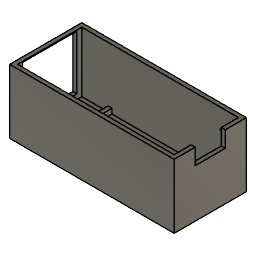
lensdisplayModule (Autodesk Fusion 360 design; units mm, degrees)
part number: 2026-07-30-17-18-59-911
part number: 2026-07-30-18-52-39-919
Autodesk Fusion 360 part; units mm, degrees
sketch "Sketch1" plane through (0, 0, 0) normal (0, 1, 0) x (1, 0, 0) in component "Display_Lens"
sketch "Sketch2" plane through (0, 0, 0) normal (0, 0, 1) x (1, 0, 0) in component "Display_Lens"
  line L0 (0, 0) -> (82, 0)
  line L1 (82, 0) -> (82, 36)
  line L2 (82, 36) -> (0, 36)
  line L3 (0, 36) -> (0, 0)
  dimension "d1" = 82
  dimension "d2" = 36
  constraint horizontal L0
  constraint vertical L1
  constraint horizontal L2
  constraint vertical L3
  constraint coincident L0.start L3.end
  measures "d1" distance of L0.start L0.end
  measures "d2" distance of L0.start L2.end
extrude "ExtrudedCentralBase" add sketch "Sketch2" along normal blind 34 in component "Display_Lens"
shell "Removed2mmTop" thickness 2 removed faces 1 at (27.3333, 24, 34) in component "Display_Lens"
sketch "CreatedLensViewWindow" plane through (2, 0, 0) normal (1, 0, 0) x (0, 1, 0) in component "Display_Lens"
  line L0 (2, 2) -> (34, 2)
  line L1 (34, 2) -> (34, 34)
  line L2 (34, 34) -> (2, 34)
  line L3 (2, 34) -> (2, 2)
  line L4 (4.5, 31.5) -> (31.5, 31.5)
  line L5 (31.5, 31.5) -> (31.5, 4.5)
  line L6 (31.5, 4.5) -> (4.5, 4.5)
  line L7 (4.5, 4.5) -> (4.5, 31.5)
  line L8 (4.5, 31.5) -> (31.5, 4.5) construction
  line L9 (31.5, 31.5) -> (4.5, 4.5) construction
  point P0 (18, 18)
  dimension "d8" = 27
  dimension "d9" = 27
  constraint horizontal L4
  constraint perpendicular L4 L5
  constraint parallel L4 L6
  constraint parallel L5 L7
  constraint coincident L8 P0
  constraint coincident L9 P0
  measures "d8" distance of L5.end L6.end
  measures "d9" distance of L4.end L5.end
extrude "ExtrudeOledViewWindow" cut sketch "CreatedLensViewWindow" against normal blind 2 contours L4 L5 L6 L7 in component "Display_Lens"
sketch "CreatedOledBackHold" plane through (0, 0, 2) normal (0, 0, 1) x (-1, 0, 0) in component "Display_Lens"
  line L0 (-2, -34) -> (-2, -2)
  line L1 (-2, -2) -> (-80, -2)
  line L2 (-80, -2) -> (-80, -34)
  line L3 (-80, -34) -> (-2, -34)
  line L4 (-17, -2) -> (-15, -2)
  line L5 (-15, -2) -> (-15, -34)
  line L6 (-15, -34) -> (-17, -34)
  line L7 (-17, -34) -> (-17, -2)
  constraint horizontal L4
  constraint vertical L5
  constraint horizontal L6
  constraint vertical L7
  constraint coincident L3 L5.end
  constraint coincident L1 L4.start
extrude "ExtrudeOledBackHold" add sketch "CreatedOledBackHold" along normal blind 2.5 contours L1 L3 L4 L5 L6 L7 in component "Display_Lens"
sketch "ConstructCableSpace" plane through (82, 0, 0) normal (1, 0, 0) x (0, 1, 0) in component "Display_Lens"
  line L0 (0, 0) -> (36, 0)
  line L1 (36, 0) -> (36, 34)
  line L2 (36, 34) -> (0, 34)
  line L3 (0, 34) -> (0, 0)
  line L4 (10.5, 34) -> (25.5, 34)
  line L5 (25.5, 34) -> (25.5, 24)
  line L6 (25.5, 24) -> (10.5, 24)
  line L7 (10.5, 24) -> (10.5, 34)
  dimension "d14" = 15
  dimension "d15" = 10
  constraint horizontal L4
  constraint vertical L5
  constraint horizontal L6
  constraint vertical L7
  constraint collinear L2 L4
  measures "d14" distance of L4.start L4.end
  measures "d15" distance of L4.start L6.end
extrude "MadeCableSpace" cut sketch "ConstructCableSpace" against normal blind 2 contours L2 L4 L5 L6 L7 in component "Display_Lens"
extrude "MadeTop2mmSmaller" cut 1 faces at (28, 0.6667, 34) along direction (0, 0, -1) blind 2 in component "Display_Lens"
sketch "CreateOledHolder" plane through (0, 0, 2) normal (0, 0, 1) x (-1, 0, 0) in component "Display_Lens"
  line L0 (-17, -34) -> (-17, -2)
  line L1 (-17, -2) -> (-80, -2)
  line L2 (-80, -2) -> (-80, -34)
  line L3 (-80, -34) -> (-17, -34)
  line L4 (-77, -28) -> (-75, -28)
  line L5 (-75, -28) -> (-75, -8)
  line L6 (-75, -8) -> (-77, -8)
  line L7 (-77, -8) -> (-77, -28)
  dimension "d23" = 3
  constraint horizontal L4
  constraint vertical L5
  constraint horizontal L6
  constraint vertical L7
  measures "d23" distance of L2 L7
extrude "ExtrudeOledHolder" add sketch "CreateOledHolder" along normal blind 3 contours L4 L5 L6 L7 in component "Display_Lens"
sketch "MadeFirstNotch" plane through (80, 0, 0) normal (-1, 0, 0) x (0, -1, 0) in component "Display_Lens"
  line L0 (-25.5, 32) -> (-34, 32)
  line L1 (-34, 32) -> (-34, 2)
  line L2 (-34, 2) -> (-2, 2)
  line L3 (-2, 2) -> (-2, 32)
  line L4 (-2, 32) -> (-10.5, 32)
  line L5 (-10.5, 32) -> (-10.5, 24)
  line L6 (-10.5, 24) -> (-25.5, 24)
  line L7 (-25.5, 24) -> (-25.5, 32)
  line L8 (-28.8, 28.8) -> (-28, 28.8)
  line L9 (-28, 28.8) -> (-28, 28)
  line L10 (-28, 28) -> (-28.8, 28)
  line L11 (-28.8, 28) -> (-28.8, 28.8)
  dimension "d26" = 0.8
  dimension "d27" = 0.8
  dimension "d29" = 5.2
  dimension "d43" = 3.2
  constraint horizontal L8
  constraint vertical L9
  constraint horizontal L10
  constraint vertical L11
  measures "d26" distance of L8.start L8.end
  measures "d27" distance of L8.start L10.end
  measures "d29" distance of L1 L11
  measures "d43" distance of L0 L8
extrude "ExtrudeFirstNotch" add sketch "MadeFirstNotch" along normal blind 3 contours L8 L9 L10 L11 in component "Display_Lens"
sketch "madeSecondNotch" plane through (80, 0, 0) normal (-1, 0, 0) x (0, -1, 0) in component "Display_Lens"
  line L0 (-28.8, 28) -> (-28.8, 28.8)
  line L1 (-28.8, 28.8) -> (-28, 28.8)
  line L2 (-28, 28.8) -> (-28, 28)
  line L3 (-28, 28) -> (-28.8, 28)
  line L4 (-25.5, 32) -> (-34, 32)
  line L5 (-34, 32) -> (-34, 2)
  line L6 (-34, 2) -> (-2, 2)
  line L7 (-2, 2) -> (-2, 32)
  line L8 (-2, 32) -> (-10.5, 32)
  line L9 (-10.5, 32) -> (-10.5, 24)
  line L10 (-10.5, 24) -> (-25.5, 24)
  line L11 (-25.5, 24) -> (-25.5, 32)
  line L12 (-8, 28.8) -> (-7.2, 28.8)
  line L13 (-7.2, 28.8) -> (-7.2, 28)
  line L14 (-7.2, 28) -> (-8, 28)
  line L15 (-8, 28) -> (-8, 28.8)
  dimension "d32" = 0.8
  dimension "d33" = 0.8
  dimension "d35" = 5.2
  dimension "d42" = 3.2
  constraint horizontal L12
  constraint vertical L13
  constraint horizontal L14
  constraint vertical L15
  measures "d32" distance of L12.start L12.end
  measures "d33" distance of L12.start L14.end
  measures "d35" distance of L7 L13
  measures "d42" distance of L8 L12
extrude "ExtrudeSecondNotch" add sketch "madeSecondNotch" along normal blind 3 contours L12 L13 L14 L15 in component "Display_Lens"
component "Display_Lens" placed x (1, 0, 0) y (0, 1, 0) z (0, 0, 1) at (0, 0, 0)
equation "OledCapsule = 3 mm" comment "3 mm from back inner plane, 20 mm in length, 2mm in width, 3mm height"
equation "SmallNothesOLED = 0.8 mm" comment "0.8X0.8 NOTHES. 5.2 from left side of inner wall, 5.2 considering outer high wall"
equation "DisplayLensDistance = 65 mm" comment "Distance from inner back wall to inner(front) lens holder"
equation "WallsThickness = 2 mm"
equation "LensOpening = 27 mm" comment "27Width27.5Height"
equation "LensHolderOffset = 13 mm" comment "Offset considerign inner front wall and inner holder wall"
